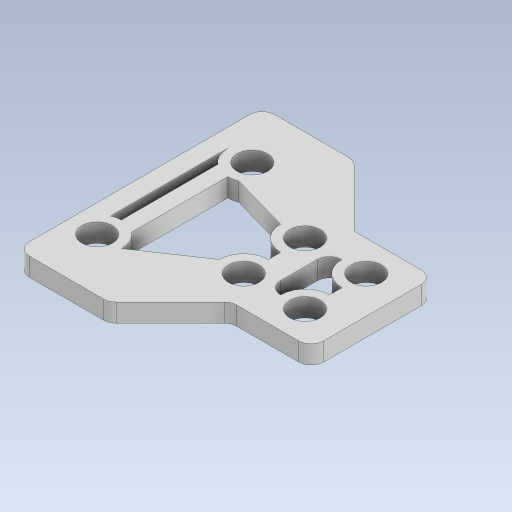
# Autodesk Inventor part: Base
Saved by Autodesk Inventor 2023.5 (Build 275446000, 446)
## iProperties
Created: 2025-10-05
Part Number: Base
Material: Generic
Document SubType Name: Modeling
Designer: Guntur
Density: 1 g/cm^3
Appearance: Default
Author: Guntur
## iProperties of the stored document Base_3DPrint.ipt
Created: 2025-10-05
Part Number: Base_3DPrint
Material: Generic
Document SubType Name: Modeling
Designer: Guntur
Density: 1 g/cm^3
Appearance: Default
Author: Guntur
Autodesk Inventor part; units mm, degrees
ref_plane "YZ Plane" through (0, 0, 0) normal (1, 0, 0) x (0, 1, 0)
ref_plane "XZ Plane" through (0, 0, 0) normal (0, 1, 0) x (-1, 0, 0)
ref_plane "XY Plane" through (0, 0, 0) normal (0, 0, 1) x (1, 0, 0)
sketch "Sketch1" plane through (0, 0, 0) normal (0, 1, 0) x (-1, 0, 0)
  line L0 (16, 0) -> (-17, 0) construction
  line L1 (0, 17) -> (0, -22.3854) construction
  circle A0 centre (0, -11.4) radius 2.5
  line L2 (18, 20) -> (-18, 20)
  line L3 (-18, 20) -> (-18, -20)
  line L4 (-18, -20) -> (18, -20)
  line L5 (18, -20) -> (18, 20)
  line L6 (18, 20) -> (-18, -20) construction
  line L7 (-18, 20) -> (18, -20) construction
  circle A1 centre (-15, 5) radius 2.5
  circle A2 centre (-15, -5) radius 2.5
  line L8 (0, 20) -> (7, 20)
  line L9 (7, 20) -> (7, -20)
  line L10 (7, -20) -> (0, -20)
  line L11 (0, -20) -> (0, 20)
  line L12 (-18, 20) -> (-8, 20)
  line L13 (-8, 20) -> (-18, 10)
  line L14 (-8, -20) -> (-18, -10)
  circle A3 centre (0, -11.4) radius 4
  circle A4 centre (-15, 5) radius 1.5183
  circle A5 centre (-15, 5) radius 4
  circle A6 centre (-15, -5) radius 4
  line L15 (-15, 1) -> (-15, -1)
  line L16 (-18, 10) -> (-31, 10)
  line L17 (-31, 10) -> (-31, -10)
  line L18 (-31, -10) -> (-18, -10)
  line L19 (-18, -10) -> (-18, 10)
  circle A7 centre (-25, -5) radius 2.5
  circle A8 centre (-25, -5) radius 4
  circle A9 centre (-25, 5) radius 2.5
  circle A10 centre (-25, 5) radius 4
  line L20 (-19, 5) -> (-21, 5)
  line L21 (-25, 1) -> (-25, -1)
  line L22 (-21, -5) -> (-19, -5)
  line L23 (-19, 5) -> (-19, -5)
  circle A11 centre (2.5, 11.4) radius 2.5
  circle A12 centre (2.5, 11.4) radius 4
  line L24 (2.5674, -8.3326) -> (2.5674, 7.4006)
  line L25 (4, -11.4) -> (4, 7.6919)
  line L26 (-11, 5) -> (-1.5, 11.4)
  line L27 (-1.5, -7.6919) -> (-11, -5)
  point P0 (0, 0)
  point P1 (-13.4817, 5)
  point P2 (-4, -11.4)
  point P3 (-15.4402, 3.5469)
  point P4 (2.5674, 8.3326)
  point P5 (0, -7.4)
  point P6 (-11, -5)
  point P7 (1.9692, -7.9183)
  point P8 (0, -15.4)
  point P9 (0, 8.2775)
  point P10 (-18, 2.3542)
  point P11 (-18, -2.3542)
  point P12 (-18, -7.6458)
  point P13 (-18, 7.6458)
  dimension "d2" = 36
  dimension "d3" = 40
  dimension "d4" = 5
  dimension "d6" = 5
  dimension "d8" = 10
  dimension "d9" = 45
  dimension "d13" = 8
  dimension "d15" = 8
  dimension "d16" = 8
  dimension "d17" = 13
  dimension "d18" = 5
  dimension "d19" = 10
  dimension "d20" = 8
  dimension "d22" = 5
  dimension "d23" = 4.5
  dimension "d24" = 8
  constraints: 56 end point, 21 point on circle, 13 centre point, 8 parallel, 7 coincident, 6 perpendicular, 5 horizontal, 5 symmetric about line, 3 midpoint, 3 point on line, 3 vertical, 1 tangent, 4 other
  measures "d2" distance of L4.end L3.end
  measures "d3" distance of L3.end L2.end
  measures "d4" diameter of A1
  measures "d6" distance from line of L0 A1.centre
  measures "d8" distance of L2.end L12.end
  measures "d9" angle of L12 L13
  measures "d13" diameter of A3
  measures "d15" diameter of A5
  measures "d16" diameter of A6
  measures "d17" distance of L18.end L17.end
  measures "d18" diameter of A7
  measures "d19" distance of A7.centre A2.centre
  measures "d20" diameter of A8
  measures "d22" diameter of A11
  measures "d23" distance from line of L9 A11.centre
  measures "d24" diameter of A12
extrude "Extrusion1" add sketch "Sketch1" along normal blind 3 contours A0 L11 A3 | A0 L11 A3 | L11 A12 L24 A3 | A3 L25 A12 L11 L2 L9 L4 | L11 L4 L14 L3 A6 L27 A3 | A12 L11 | L11 A12 | L26 A5 L3 L13 L2 L11 A12 | A6 L3 | A5 L3 | A6 L3 A5 L15 | A6 L3 | L3 L18 L17 L16 A5 L20 A10 L21 A8 L22 A6 | L3 A5 | A6 L23 A5 L3 | A8 | A10
fillet "Fillet1" radius 2 9 edges at (18, 1.5, 10) (8, 1.5, -20) (-7, 1.5, -20) (-7, 1.5, 20) (8, 1.5, 20) (31, 1.5, 10) (31, 1.5, -10) (19, 1.5, 5) (19, 1.5, -5)
body "Solid1"
